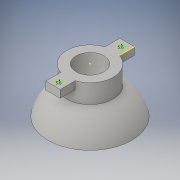
# Autodesk Inventor part: Vacuum Gripper
Saved by Autodesk Inventor 2016 (Build 200138000, 138)
## iProperties
Created: 2017-10-11
Part Number: Vacuum Gripper
Material: Generic
Document SubType Name: Modeling
Designer: ls769
Density: 1 g/cm^3
Appearance: Default
Author: ls769
Autodesk Inventor part; units mm, degrees
ref_plane "YZ Plane" through (0, 0, 0) normal (1, 0, 0) x (0, 1, 0)
ref_plane "XZ Plane" through (0, 0, 0) normal (0, 1, 0) x (-1, 0, 0)
ref_plane "XY Plane" through (0, 0, 0) normal (0, 0, 1) x (1, 0, 0)
sketch "Sketch1" plane through (0, 0, 0) normal (0, 0, 1) x (1, 0, 0)
  line L0 (22.5, 44) -> (22.5, 25.6111)
  line L1 (13.5, 44) -> (13.5, 29.9618)
  arc A0 (22.5, 18.6538) -> (13.5, 23.9242) centre (0, -9.4487) ccw
  arc A1 (34.7379, 0) -> (22.5, 18.6538) centre (0, -9.4487) ccw
  arc A2 (40.5729, 0) -> (22.5, 25.6111) centre (0, -9.4487) ccw
  line L2 (13.5, 29.9618) -> (13.5, 23.9242)
  line L3 (13.5, 44) -> (22.5, 44)
  line L4 (34.7379, 0) -> (40.5729, 0)
  line L5 (0, -20.1384) -> (0, 54.6897) projected
  point P0 (0, 0)
  constraints: 10 end point, 6 point on circle, 3 centre point, 1 coincident, 1 horizontal, 1 parallel
revolve "Revolution1" add sketch "Sketch1" angle 360 about axis through (0, -10, 0) along (0, 1, 0)
sketch "Sketch2" plane through (0, 44, 0) normal (0, 1, 0) x (1, 0, 0)
  line L0 (-7, -13.5) -> (-7, -36)
  line L1 (-7, -36) -> (7, -36)
  line L2 (7, -36) -> (7, -13.5)
  line L3 (7, -13.5) -> (7, -11.5434)
  circle A0 centre (0, 0) radius 13.5 projected
  line L4 (-7, -13.5) -> (-7, -11.5434)
  line L5 (-7, 13.5) -> (-7, 36)
  line L6 (-7, 36) -> (7, 36)
  line L7 (7, 36) -> (7, 13.5)
  line L8 (-7, 13.5) -> (-7, 11.5434)
  line L9 (7, 13.5) -> (7, 11.5434)
  dimension "d12" = 14
  dimension "d13" = 22.5
  dimension "d16" = 14
  dimension "d17" = 22.5
  constraints: 20 end point, 4 parallel, 4 point on circle, 2 vertical
  measures "d12" distance of L1.end L0.end
  measures "d13" distance of L0.end L0.start
  measures "d16" distance of L5.end L6.end
  measures "d17" distance of L5.start L5.end
extrude "Extrusion1" add sketch "Sketch2" against normal blind 7.5 contours L4 A0 L3 L2 L1 L0 | L8 L5 L6 L7 L9 A0
sketch "Sketch3" plane through (-7, 44, -36) normal (0, 1, 0) x (1, 0, 0)
  circle A0 centre (7, -66.0778) radius 2.8
  circle A1 centre (7.0706, -5.9222) radius 2.8
  line L0 (14, -14.6166) -> (14, 0) projected
  point P0 (7, -36)
  dimension "d20" = 5.6
  dimension "d21" = 5.6
  constraints: 2 centre point
  measures "d20" diameter of A0
  measures "d21" diameter of A1
body "Solid1"
